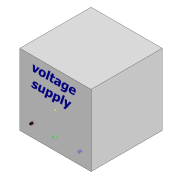
# Autodesk Inventor part: voltage_supply
Saved by Autodesk Inventor 2021 (Build 250183000, 183)
## iProperties
Created: 2022-02-10
Part Number: voltage_supply
Material: Типовые
Document SubType Name: Modeling
Designer: Тиннелла о Каллинике
Density: 1 g/cm^3
Appearance: По умолчанию
Author: Тиннелла о Каллинике
Autodesk Inventor part; units mm, degrees
ref_plane "YZ Plane" through (0, 0, 0) normal (1, 0, 0) x (0, 1, 0)
ref_plane "XZ Plane" through (0, 0, 0) normal (0, 1, 0) x (-1, 0, 0)
sketch "Эскиз1" plane through (0, 0, 0) normal (0, 0, 1) x (1, 0, 0)
  line L0 (-5, 5) -> (5, 5)
  line L1 (5, 5) -> (5, -5)
  line L2 (5, -5) -> (-5, -5)
  line L3 (-5, -5) -> (-5, 5)
  point P0 (0, 0)
  point P1 (5, 0)
  point P2 (0, 5)
  dimension "d0" = 10
  dimension "d1" = 10
  constraints: 8 end point, 2 midpoint, 2 parallel, 1 horizontal, 1 horizontal alignment, 1 perpendicular, 1 vertical alignment
  measures "d0" distance of L0.end L1.end
  measures "d1" distance of L0.start L0.end
extrude "Выдавливание1" add sketch "Эскиз1" against normal blind 10
sketch "Эскиз2" plane through (0, 0, 0) normal (0, 0, 1) x (1, 0, 0)
  line L0 (-3.4766, 4.33) -> (6.5107, 4.33) construction
  line L1 (6.5107, 4.33) -> (6.5107, 1.2958) construction
  line L2 (6.5107, 1.2958) -> (-3.4766, 1.2958) construction
  line L3 (-3.4766, 1.2958) -> (-3.4766, 4.33) construction
  point P0 (0, 0)
  constraints: 2 other
ref_plane "РабПлоскость1" through (0, 0, 0) normal (0, 0, 1) x (1, 0, 0)
sketch "Эскиз3" plane through (0, 0, 0) normal (0, 0, 1) x (1, 0, 0)
  circle A0 centre (-3.2379, -3.1898) radius 0.15
  point P0 (0, 0)
  dimension "d5" = 0.3
  constraints: 1 centre point
  measures "d5" diameter of A0
extrude "Выдавливание2" add sketch "Эскиз3" along normal blind 0.3 separate body
sketch "Эскиз4" plane through (0, 0, 0) normal (0, 0, 1) x (1, 0, 0)
  circle A0 centre (0, -3.1898) radius 0.15
  point P0 (0, 0)
  dimension "d10" = 0.3
  constraints: 1 centre point
  measures "d10" diameter of A0
extrude "Выдавливание3" add sketch "Эскиз4" along normal blind 0.3 separate body
sketch "Эскиз5" plane through (0, 0, 0) normal (0, 0, 1) x (1, 0, 0)
  circle A0 centre (3.5688, -3.1898) radius 0.15
  point P0 (0, 0)
  dimension "d13" = 0.3
  constraints: 1 centre point
  measures "d13" diameter of A0
extrude "Выдавливание4" add sketch "Эскиз5" along normal blind 0.3 separate body
